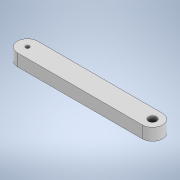
# Autodesk Inventor part: push_rod
Saved by Autodesk Inventor 2020 (Build 240168000, 168)
## iProperties
Created: 2020-07-26
Part Number: push_rod
Material: Generic
Document SubType Name: Modeling
Designer: Aarya
Density: 1 g/cm^3
Appearance: Default
Author: Aarya
Autodesk Inventor part; units mm, degrees
ref_plane "YZ Plane" through (0, 0, 0) normal (1, 0, 0) x (0, 1, 0)
ref_plane "XZ Plane" through (0, 0, 0) normal (0, 1, 0) x (-1, 0, 0)
ref_plane "XY Plane" through (0, 0, 0) normal (0, 0, 1) x (1, 0, 0)
sketch "Sketch1" plane through (0, 0, 0) normal (0, 1, 0) x (-1, 0, 0)
  line L0 (15.5, 2.5) -> (-15.5, 2.5)
  line L1 (-18, 0) -> (-18, 0)
  line L2 (-15.5, -2.5) -> (15.5, -2.5)
  line L3 (18, 0) -> (18, 0)
  line L4 (18, 2.5) -> (-18, -2.5) construction
  line L5 (-18, 2.5) -> (18, -2.5) construction
  arc A0 (18, 0) -> (15.5, 2.5) centre (15.5, 0) ccw
  arc A1 (15.5, -2.5) -> (18, 0) centre (15.5, 0) ccw
  arc A2 (-15.5, 2.5) -> (-18, 0) centre (-15.5, 0) ccw
  arc A3 (-18, 0) -> (-15.5, -2.5) centre (-15.5, 0) ccw
  circle A4 centre (15.5, 0) radius 0.475
  circle A5 centre (-15.5, 0) radius 1
  point P0 (0, 0)
  point P1 (-18, 0)
  point P2 (18, 0)
  dimension "d0" = 5
  dimension "d1" = 2.5
  dimension "d2" = 31
  dimension "d3" = 0.95
  dimension "d4" = 2
  constraints: 12 end point, 8 point on circle, 8 point on line, 8 tangent, 6 centre point, 3 equal radius, 2 coincident, 2 midpoint, 2 parallel, 1 horizontal, 1 perpendicular
  measures "d0" distance of L5.end L4.start
  measures "d1" radius of A0
  measures "d2" distance of L0.start L0.end
  measures "d3" diameter of A4
  measures "d4" diameter of A5
extrude "Extrusion1" add sketch "Sketch1" along normal blind 3
body "Solid1"
